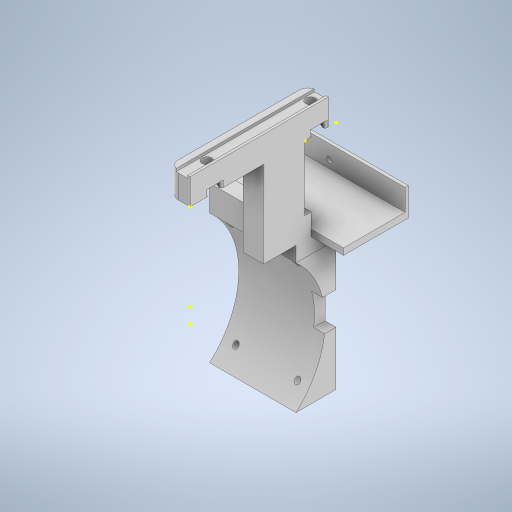
# Autodesk Inventor part: Back
Saved by Autodesk Inventor 2024 (Build 280153000, 153)
## iProperties
Created: 2023-12-18
Part Number: Back
Material: Generic
Document SubType Name: Modeling
Designer: Mechatronics Lab 1
Density: 1 g/cm^3
Appearance: Default
Author: Mechatronics Lab 1
Autodesk Inventor part; units mm, degrees
ref_plane "YZ Plane" through (0, 0, 0) normal (1, 0, 0) x (0, 1, 0)
ref_plane "XZ Plane" through (0, 0, 0) normal (0, 1, 0) x (-1, 0, 0)
ref_plane "XY Plane" through (0, 0, 0) normal (0, 0, 1) x (1, 0, 0)
sketch "Sketch1" plane through (0, 0, 0) normal (0, 1, 0) x (-1, 0, 0)
  line L0 (0, 0) -> (9.5, 0)
  line L1 (9.5, 0) -> (9.5, -64)
  line L2 (9.5, -64) -> (0, -64)
  line L3 (0, -64) -> (0, 0)
  circle A0 centre (3.7, -11.5) radius 2.25
  circle A1 centre (3.7, -59.5) radius 2.25
  line L4 (3.7, -11.5) -> (3.7, -59.5) construction
  dimension "d1" = 9.5
  dimension "d2" = 64
  dimension "d3" = 4.5
  dimension "d4" = 48
  dimension "d6" = 3.7
  dimension "d17" = 4.5
  constraints: 10 end point, 2 centre point, 2 parallel, 1 equal radius, 1 horizontal, 1 perpendicular, 1 vertical
  measures "d1" distance of L0.start L0.end
  measures "d2" distance of L0.end L1.end
  measures "d3" diameter of A0
  measures "d4" distance of L4.start L4.end
  measures "d6" distance between parallel lines of L3 L4
  measures "d17" distance from line of L4.end L2
extrude "Extrusion1" add sketch "Sketch1" along normal blind 12
sketch "Sketch2" plane through (-9.5, 0, 0) normal (0, 0, 1) x (1, 0, 0)
  line L0 (9.5, 12) -> (0, 12) projected
  line L1 (3, 12) -> (8.4, 12)
  line L2 (8.4, 12) -> (8.4, 10.8)
  line L3 (8.4, 10.8) -> (3, 10.8)
  line L4 (3, 10.8) -> (3, 12)
  line L5 (9.5, 0) -> (9.5, 12) projected
  line L6 (3.55, 0) -> (8.05, 0) projected
  line L7 (3.55, 12) -> (8.05, 12) projected
  line L8 (9.5, 0) -> (9.5, 12) projected
  line L9 (9.5, 0) -> (9.5, 12) projected
  line L10 (3.55, 12) -> (8.05, 12) projected
  line L11 (3.55, 12) -> (3.55, 0) projected
  line L12 (3.55, 12) -> (8.05, 12) projected
  line L13 (3.55, 0) -> (8.05, 0) projected
  line L14 (3.55, 12) -> (8.05, 12) projected
  line L15 (3.55, 0) -> (8.05, 0) projected
  line L16 (3.55, 12) -> (8.05, 12) projected
  line L17 (3.55, 0) -> (8.05, 0) projected
  dimension "d9" = 1.1
  dimension "d10" = 5.4
  dimension "d11" = 1.2
  dimension "d76" = 12
  constraints: 8 end point, 2 parallel, 1 horizontal, 1 perpendicular, 1 point on line
  measures "d9" distance between parallel lines of L5 L2
  measures "d10" distance of L2.end L3.end
  measures "d11" distance between parallel lines of L0 L3
  measures "d76" distance between parallel lines of L6 L7
extrude "Extrusion2" cut sketch "Sketch2" against normal up to next
sketch "Sketch3" plane through (0, 0, 0) normal (0, -1, 0) x (1, 0, 0)
  circle A0 centre (-3.7, -11.5) radius 2.25 projected
  circle A1 centre (-3.7, -11.5) radius 3.75
  circle A2 centre (-3.7, -59.5) radius 2.25 projected
  circle A3 centre (-3.7, -59.5) radius 3.75
  point P0 (0, 0)
  dimension "d14" = 7.5
  constraints: 2 centre point, 2 coincident, 1 equal radius
  measures "d14" diameter of A3
extrude "Extrusion3" cut sketch "Sketch3" against normal blind 3
fillet "Fillet1" radius 1 4 edges at (0, 1.5, -58.8897) (0, 1.5, -60.1103) (0, 1.5, -10.8897) (0, 1.5, -12.1103)
fillet "Fillet2" radius 4 2 edges at (-9.5, 6, -64) (-9.5, 6, 0)
sketch "Sketch28" plane through (0, 0, 0) normal (0, -1, 0) x (1, 0, 0)
  arc A0 (-1.5684, -56.4147) -> (0, -55.592) centre (-1, -55.592) ccw projected
  line L0 (0, -55.592) -> (0, -53)
  line L1 (0, -15.408) -> (0, -55.592) projected
  line L2 (-9.5, -60) -> (-9.5, -4) projected
  line L3 (0, -53) -> (-9.5, -53)
  line L4 (-9.5, -53) -> (-9.5, -34)
  line L5 (-9.5, -34) -> (0, -34)
  line L6 (0, -34) -> (0, -53)
  point P0 (0, 0)
  point P1 (0, -34)
  dimension "d107" = 2.592
  dimension "d108" = 19
  constraints: 10 end point, 2 parallel, 2 point on line, 1 horizontal, 1 perpendicular
  measures "d107" distance of L0.start L0.end
  measures "d108" distance of L3.end L4.end
extrude "Extrusion19" add sketch "Sketch28" along normal blind 30
sketch "Sketch40" plane through (0, -30, 0) normal (0, -1, 0) x (1, 0, 0)
  line L0 (0, -53) -> (-9.5, -53) projected
  line L1 (-9.5, -53) -> (-9.5, -56)
  line L2 (-9.5, -56) -> (0, -56)
  line L3 (0, -56) -> (0, -34)
  line L4 (0, 0) -> (0, -64) projected
  line L5 (0, -34) -> (-9.5, -34)
  line L6 (-9.5, -34) -> (-9.5, -53)
  line L7 (-9.5, -34) -> (0, -34)
  line L8 (0, -34) -> (0, -56)
  line L9 (0, -56) -> (-9.5, -56)
  line L10 (-9.5, -56) -> (-9.5, -34)
  dimension "d130" = 3
  dimension "d131" = 22
  constraints: 18 end point, 3 perpendicular, 2 parallel, 2 point on line, 1 collinear, 1 horizontal, 1 vertical
  measures "d130" distance of L0.end L1.end
  measures "d131" distance of L2.end L3.end
extrude "Extrusion21" add sketch "Sketch40" along normal blind 10
sketch "Sketch41" plane through (0, 0, -53) normal (0, 0, -1) x (-1, 0, 0)
  point P0 (0, 0)
sketch "Sketch42" plane through (0, -40, 0) normal (0, -1, 0) x (1, 0, 0)
  line L0 (-9.5, -56) -> (0, -56) projected
  line L1 (-9.5, -56) -> (-40, -56)
  line L2 (-9.5, -56) -> (21, -56) construction
  line L3 (-40, -56) -> (-40, -49)
  line L4 (-40, -49) -> (0, -49)
  line L5 (0, -49) -> (0, -56)
  line L6 (0, -56) -> (-9.5, -56)
  point P0 (0, 0)
  point P1 (0, -56)
  dimension "d134" = 30.5
  dimension "d135" = 180
  dimension "d136" = 7
  dimension "d137" = 40
  dimension "d138" = 7
  constraints: 12 end point, 2 horizontal, 2 perpendicular, 1 collinear, 1 point on line
  measures "d134" distance of L0.start L1.end
  measures "d135" angle of L1 L2
  measures "d136" distance of L1.end L3.end
  measures "d137" distance of L3.end L4.end
  measures "d138" distance of L4.end L5.end
extrude "Extrusion22" add sketch "Sketch42" along normal blind 7
sketch "Sketch54" plane through (-40, -40, -56) normal (-1, 0, 0) x (0, 0, 1)
  arc A0 (7, -7) -> (7, -57) centre (31.4949, -32) ccw projected
  line L0 (-6.4428, -57) -> (19.2704, -57)
  line L1 (19.2704, -57) -> (19.2704, -74.6848)
  line L2 (19.2704, -74.6848) -> (-6.4428, -74.6848)
  line L3 (-6.4428, -74.6848) -> (-6.4428, -57)
  point P0 (56, 40)
  constraints: 8 end point, 2 parallel, 1 horizontal, 1 perpendicular
extrude "Extrusion25" cut sketch "Sketch54" against normal blind 104.3
sketch "Sketch56" plane through (0, -47, 0) normal (0, -1, 0) x (1, 0, 0)
  line L0 (-40, -56) -> (0, -56) projected
  line L1 (0, -56) -> (0, -49) projected
  line L2 (-40, -56) -> (0, -56)
  line L3 (0, -56) -> (0, -49)
  line L4 (0, -49) -> (-40, -49)
  line L5 (-40, -49) -> (-40, -56)
  point P0 (0, 0)
  point P1 (9.3, -58)
  constraints: 8 end point, 2 parallel, 1 horizontal, 1 perpendicular, 2 other
sketch "Sketch58" plane through (-40, -40, -56) normal (-1, 0, 0) x (0, 0, 1)
  arc A0 (7, -7) -> (7, -67) centre (33.4575, -37) ccw
  point P0 (56, 40)
  dimension "d164" = 60
  dimension "d165" = 40
  constraints: 2 point on circle, 1 centre point
  measures "d164" distance of A0.start A0.end
  measures "d165" radius of A0
sweep "Sweep4" add profiles "Sketch56" path "Sketch58" separate body
sketch "Sketch59" plane through (-40, -47, -56) normal (-1, 0, 0) x (0, 0, 1)
  line L0 (7.875, -66.9451) -> (7, -60) projected
  line L1 (7, -60) -> (-3.876, -60)
  line L2 (-3.876, -60) -> (-3.876, -70.2842)
  line L3 (-3.876, -70.2842) -> (7, -70.2842)
  line L4 (7, -70.2842) -> (7, -60)
  line L5 (-3.876, -60) -> (12.796, -60)
  line L6 (12.796, -60) -> (12.796, -72.0421)
  line L7 (12.796, -72.0421) -> (-3.876, -72.0421)
  line L8 (-3.876, -72.0421) -> (-3.876, -60)
  point P0 (56, 47)
  point P1 (7, -60)
  constraints: 16 end point, 4 parallel, 2 horizontal, 2 perpendicular
extrude "Extrusion26" cut sketch "Sketch59" against normal blind 63.025 bodies 2
sketch "Sketch60" plane through (0, -40, 0) normal (0, 1, 0) x (1, 0, 0)
  point P0 (0, 0)
sketch "Sketch61" plane through (-40, -47, -56) normal (-1, 0, 0) x (0, 0, 1)
  arc A0 (0, 0) -> (0, -60) centre (33.4575, -30) ccw projected
  line L0 (-11.4803, -30) -> (-11.4803, 0)
  line L1 (-11.4803, 0) -> (0, 0)
  line L2 (-11.4803, -30) -> (-11.4803, -60)
  line L3 (-11.4803, -60) -> (0, -60)
  arc A1 (0, 0) -> (0, -60) centre (33.4575, -30) ccw
  point P0 (56, 47)
  constraints: 8 end point, 4 point on circle, 3 tangent, 2 perpendicular, 2 vertical, 1 centre point
extrude "Extrusion27" add sketch "Sketch61" against normal blind 40 bodies 2
sketch "Sketch62" plane through (-40, -47, -49) normal (0, 1, 0) x (1, 0, 0)
  point P0 (40, -49)
sketch "Sketch63" plane through (-40, -40, -56) normal (-1, 0, 0) x (0, 0, 1)
  line L0 (0, 10) -> (0, -7) projected
  line L1 (0, -7) -> (-11.4803, -7)
  line L2 (-11.4803, -7) -> (-11.4803, 0)
  line L3 (-11.4803, 0) -> (0, 0)
  line L4 (0, 0) -> (0, -7)
  point P0 (56, 40)
  point P1 (0, 0)
  dimension "d172" = 7
  constraints: 8 end point, 2 parallel, 1 horizontal, 1 perpendicular
  measures "d172" distance of L1.end L2.end
extrude "Extrusion28" add sketch "Sketch63" against normal blind 40 bodies 1
sketch "Sketch64" plane through (0, -40, 0) normal (0, 1, 0) x (1, 0, 0)
  point P0 (0, 0)
sketch "Sketch65" plane through (-40, -107, -67.4803) normal (0, 0, -1) x (-1, 0, 0)
  line L0 (-40, 0) -> (-40, 60) projected
  line L1 (-40, 25) -> (-40, 40)
  line L2 (-40, 40) -> (-35, 40)
  line L3 (-35, 40) -> (-35, 25)
  line L4 (-35, 25) -> (-40, 25)
  point P0 (-40, 107)
  point P1 (0, 0)
  dimension "d179" = 15
  dimension "d180" = 5
  dimension "d181" = 15
  constraints: 8 end point, 2 perpendicular, 2 point on line
  measures "d179" distance of L1.start L1.end
  measures "d180" distance of L1.end L2.end
  measures "d181" distance of L2.end L3.end
extrude "Extrusion29" cut sketch "Sketch65" against normal blind 20.95 bodies 2
sketch "Sketch66" plane through (0, -107, -49) normal (1, 0, 0) x (0, 0, -1)
  point P0 (-49, 107)
sketch "Sketch67" plane through (-40, -47, -67.4803) normal (0, 0, -1) x (-1, 0, 0)
  point P0 (-40, 47)
sketch "Sketch68" plane through (0, -40, 0) normal (0, 1, 0) x (1, 0, 0)
  line L0 (0, 56) -> (-9.5, 56) projected
  line L1 (15, 56) -> (-40, 56)
  line L2 (-40, 67.4803) -> (0, 67.4803) projected
  line L3 (15, 56) -> (-40, 56)
  line L4 (-40, 56) -> (-40, 86)
  line L5 (-40, 86) -> (15, 86)
  line L6 (15, 86) -> (15, 56)
  point P0 (0, 0)
  dimension "d184" = 15
  dimension "d187" = 30
  constraints: 10 end point, 2 parallel, 1 horizontal, 1 perpendicular
  measures "d184" distance of L0.start L1.start
  measures "d187" distance of L3.end L4.end
extrude "Extrusion30" add sketch "Sketch68" along normal blind 3 bodies 1
sketch "Sketch69" plane through (0, -40, 0) normal (0, 1, 0) x (1, 0, 0)
  line L0 (-40, 49) -> (-40, 56) projected
  line L1 (-9.5, 49) -> (-9.5, 56) projected
  line L2 (-40, 49) -> (-9.5, 49)
  line L3 (-9.5, 49) -> (-9.5, 56)
  line L4 (-9.5, 56) -> (-40, 56)
  line L5 (-40, 56) -> (-40, 49)
  point P0 (0, 0)
  constraints: 8 end point, 2 parallel, 1 horizontal, 1 perpendicular
extrude "Extrusion31" add sketch "Sketch69" along normal blind 3 bodies 1
sketch "Sketch70" plane through (0, -37, 0) normal (0, 1, 0) x (1, 0, 0)
  line L0 (15, 56) -> (15, 86) projected
  line L1 (-40, 86) -> (15, 86)
  line L2 (15, 86) -> (15, 84.5)
  line L3 (15, 84.5) -> (-40, 84.5)
  line L4 (-40, 84.5) -> (-40, 86)
  point P0 (0, 0)
  dimension "d192" = 1.5
  constraints: 8 end point, 2 parallel, 1 horizontal, 1 perpendicular, 1 point on line
  measures "d192" distance of L1.end L2.end
extrude "Extrusion32" add sketch "Sketch70" along normal blind 10 bodies 1
sketch "Sketch72" plane through (-40, -107, -67.4803) normal (0, 0, -1) x (-1, 0, 0)
  line L0 (0, 60) -> (0, 0) projected
  line L1 (0, 0) -> (-1, 0)
  line L2 (-1, 0) -> (-1, 3)
  line L3 (-1, 3) -> (0, 3)
  line L4 (0, 3) -> (0, 0)
  line L5 (-1, 3) -> (-39, 3)
  line L6 (-39, 3) -> (-39, 59)
  line L7 (-39, 59) -> (-1, 59)
  line L8 (-1, 59) -> (-1, 3)
  line L9 (-1, 3) -> (-6, 3)
  line L10 (-6, 3) -> (-6, 7)
  line L11 (-6, 7) -> (-1, 7)
  line L12 (-1, 7) -> (-1, 3)
  circle A0 centre (-6, 7) radius 1.25
  line L13 (-1, 59) -> (-4.5, 59)
  line L14 (-4.5, 59) -> (-4.5, 55)
  line L15 (-4.5, 55) -> (-1, 55)
  line L16 (-1, 55) -> (-1, 59)
  circle A1 centre (-4.5, 55) radius 1.25
  line L17 (-39, 59) -> (-35.5, 59)
  line L18 (-35.5, 59) -> (-35.5, 55)
  line L19 (-35.5, 55) -> (-39, 55)
  line L20 (-39, 55) -> (-39, 59)
  circle A2 centre (-35.5, 55) radius 1.25
  line L21 (-39, 3) -> (-34.5, 3)
  line L22 (-34.5, 3) -> (-34.5, 7)
  line L23 (-34.5, 7) -> (-39, 7)
  line L24 (-39, 7) -> (-39, 3)
  circle A3 centre (-34.5, 7) radius 1.25
  point P0 (-40, 107)
  dimension "d195" = 1
  dimension "d196" = 3
  dimension "d197" = 38
  dimension "d198" = 56
  dimension "d199" = 5
  dimension "d200" = 4
  dimension "d201" = 2.5
  dimension "d202" = 3.5
  dimension "d203" = 4
  dimension "d204" = 2.5
  dimension "d205" = 3.5
  dimension "d206" = 4
  dimension "d207" = 2.5
  dimension "d208" = 4.5
  dimension "d209" = 4
  dimension "d210" = 2.5
  constraints: 48 end point, 12 parallel, 6 horizontal, 6 perpendicular, 4 centre point, 4 coincident
  measures "d195" distance of L2.end L3.end
  measures "d196" distance of L1.end L2.end
  measures "d197" distance of L6.end L7.end
  measures "d198" distance of L5.end L6.end
  measures "d199" distance of L10.end L11.end
  measures "d200" distance of L9.end L10.end
  measures "d201" diameter of A0
  measures "d202" distance of L15.end L14.end
  measures "d203" distance of L14.end L13.end
  measures "d204" diameter of A1
  measures "d205" distance of L18.end L19.end
  measures "d206" distance of L17.end L18.end
  measures "d207" diameter of A2
  measures "d208" distance of L23.end L22.end
  measures "d209" distance of L22.end L21.end
  measures "d210" diameter of A3
extrude "Extrusion33" cut sketch "Sketch72" against normal blind 71.9125 contours A0 L11 L10 | L10 L11 A0 | A3 L23 L22 | L22 L23 A3 | A1 L14 L15 | L15 L14 A1 | A2 L18 L19 | L19 L18 A2 bodies 2
sketch "Sketch73" plane through (-9.5, 0, -4) normal (-1, 0, 0) x (0, 0, 1)
  line L0 (-52, -37) -> (-52, -40) projected
  line L1 (-52, -37) -> (-45, -37)
  line L2 (-45, -37) -> (-45, -35)
  line L3 (-45, -35) -> (-52, -35)
  line L4 (-52, -35) -> (-52, -37)
  point P0 (4, 0)
  dimension "d213" = 7
  dimension "d214" = 2
  constraints: 8 end point, 2 parallel, 1 horizontal, 1 perpendicular
  measures "d213" distance of L3.end L2.end
  measures "d214" distance of L2.end L1.end
extrude "Extrusion34" add sketch "Sketch73" along normal blind 30.5 bodies 1
sketch "Sketch74" plane through (-40, -107, -49) normal (0, -1, 0) x (1, 0, 0)
  line L0 (40, 0) -> (0, 0) projected
  line L1 (0, 0) -> (0, -18.4803) projected
  line L2 (0, -18.4803) -> (40, -18.4803) projected
  line L3 (0, -18.4803) -> (40, -18.4803)
  circle A0 centre (20, -14.4803) radius 1.25
  point P0 (40, 49)
  dimension "d218" = 2.5
  constraints: 2 end point, 1 centre point, 1 collinear
  measures "d218" diameter of A0
extrude "Extrusion35" cut sketch "Sketch74" against normal blind 10 bodies 2
sketch "Sketch75" plane through (15, -40, -86) normal (0, 0, -1) x (-1, 0, 0)
  line L0 (55, 13) -> (0, 13) projected
  line L1 (55, 0) -> (55, 13) projected
  line L2 (55, 6.5) -> (35, 6.5)
  circle A0 centre (35, 6.5) radius 1.25
  point P0 (15, 40)
  dimension "d221" = 20
  dimension "d222" = 2.5
  constraints: 2 end point, 1 centre point, 1 coincident, 1 horizontal, 1 midpoint
  measures "d221" distance of L2.start L2.end
  measures "d222" diameter of A0
extrude "Extrusion36" cut sketch "Sketch75" against normal blind 10 bodies 1
body "Solid1"
body "Solid2"
